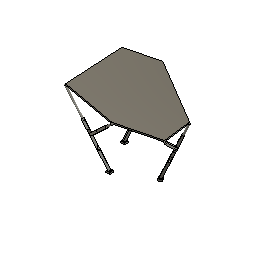
TT-5 (Autodesk Fusion 360 design; units mm, degrees)
Autodesk Fusion 360 part; units mm, degrees
sketch "Sketch1" plane through (0, 0, 0) normal (0, 1, 0) x (1, 0, 0) in component "TT-2 v5 (2)"
  line L0 (2.5, -2.5) -> (-2.5, -2.5)
  line L1 (-2.5, -2.5) -> (-2.5, 2.5)
  line L2 (-2.5, 2.5) -> (2.5, 2.5)
  line L3 (2.5, 2.5) -> (2.5, -2.5)
  constraint horizontal L0
  constraint vertical L1
  constraint horizontal L2
  constraint vertical L3
extrude "Extrude1" add sketch "Sketch1" along normal blind 2.5 makes body 1 in component "TT-2 v5 (2)"
sketch "Sketch2" plane through (0, 0, 0) normal (0, 1, 0) x (1, 0, 0) in component "TT-2 v5 (2)"
  line L0 (1.5, -1.5) -> (-1.5, -1.5)
  line L1 (-1.5, -1.5) -> (-1.5, 1.5)
  line L2 (-1.5, 1.5) -> (1.5, 1.5)
  line L3 (1.5, 1.5) -> (1.5, -1.5)
  constraint horizontal L0
  constraint vertical L1
  constraint horizontal L2
  constraint vertical L3
extrude "Extrude2" add sketch "Sketch2" along normal blind 60 separate body makes body 2 in component "TT-2 v5 (2)"
move_body "Move1" bodies 2 to x (0.939693, -0.34202, 0) y (0.34202, 0.939693, 0) z (0, 0, 1) at (-0.0905, -0.513, 0) in component "TT-2 v5 (2)"
move_body "Move2" bodies 2 to x (1, 0, 0) y (0, 1, 0) z (0, 0, 1) at (3.3727, 9.6612, 0) in component "TT-2 v5 (2)"
sphere "SpherePrimitive1" add diameter 3 placed x (0, 0, 1) y (-0.939693, 0.34202, 0) z (-0.34202, -0.939693, 0) at (3.3241, 9.1329, 0) bodies 2 in component "TT-2 v5 (2)"
sphere "SpherePrimitive2" cut diameter 3 placed x (-1, 0, 0) y (0, 0, 1) z (0, 1, 0) at (0, 2.5, 0) bodies 1 in component "TT-2 v5 (2)"
cylinder "CylinderPrimitive1" add diameter 2.5 height 40 placed x (0.883022, -0.321394, -0.34202) y (-0.321394, 0.116978, -0.939693) z (0.34202, 0.939693, 0) at (23.8453, 65.5145, 0) separate body makes body 3 in component "TT-2 v5 (2)"
sphere "SpherePrimitive3" add diameter 2.5 placed x (0, 0, -1) y (-0.939693, 0.34202, 0) z (0.34202, 0.939693, 0) at (37.5261, 103.1022, 0) bodies 3 in component "TT-2 v5 (2)"
move_body "Move3" bodies 3 2 to x (0.939693, 0.34202, 0) y (-0.34202, 0.939693, 0) z (0, 0, 1) at (23.6283, -3.8286, 0) in component "TT-2 v5 (2)"
move_body "Move4" bodies 2 3 to x (1, 0, 0) y (0, 1, 0) z (0, 0, 1) at (-23.6681, -3.196, 0) in component "TT-2 v5 (2)"
copy_body "CopyPasteBodies1" bodies 3 2 makes body 4 makes body 5 in component "TT-2 v5 (2)"
move_body "Move5" bodies 4 5 to x (1, 0, 0) y (0, 0.906308, 0.422618) z (0, -0.422618, 0.906308) at (0, 42.015, -10.6133) in component "TT-2 v5 (2)"
move_body "Move6" bodies 5 4 to x (1, 0, 0) y (0, 1, 0) z (0, 0, 1) at (0, -2.8403, 9.6134) in component "TT-2 v5 (2)"
extrude "Extrude3" cut 1 faces at (0.4157, 96.2065, 25.0427) along direction (0, -0.906308, -0.422618) blind 15 on bodies 5 bodies 5 in component "TT-2 v5 (2)"
move_body "Move7" bodies 4 to x (1, 0, 0) y (0, 1, 0) z (0, 0, 1) at (0, -26.7116, -12.4558) in component "TT-2 v5 (2)"
move_body "Move8" bodies 5 4 to x (1, 0, 0) y (0, 1, 0) z (0, 0, 1) at (0, -15.5908, 0) in component "TT-2 v5 (2)"
copy_body "CopyPasteBodies2" bodies 4 5 makes body 6 makes body 7 in component "TT-2 v5 (2)"
move_body "Move9" bodies 6 7 to x (0, 0, -1) y (0, 1, 0) z (1, 0, 0) at (-0.0791, 0, -0.06) in component "TT-2 v5 (2)"
move_body "Move10" bodies 6 to x (1, 0, 0) y (0, 1, 0) z (0, 0, 1) at (5.2397, 11.2365, 0) in component "TT-2 v5 (2)"
move_body "Move11" bodies 7 3 4 2 5 6 to x (1, 0, 0) y (0, 0.984808, -0.173648) z (0, 0.173648, 0.984808) at (0, 0.0409, 0.4679) in component "TT-2 v5 (2)"
move_body "Move12" bodies 5 4 to x (1, 0, 0) y (0, 1, 0) z (0, 0, 1) at (0, 17.3834, -3.0131) in component "TT-2 v5 (2)"
sketch "Sketch7" plane through (0, 0, 0) normal (0, 1, 0) x (1, 0, 0) in component "TT-2 v5 (2)"
  line L0 (20, -30) -> (50, 15)
  line L1 (50, 15) -> (20, 47.2574)
  line L2 (20, 47.2574) -> (-26.886, 18.4817)
  line L3 (-26.886, 18.4817) -> (-3.443, -34.2088)
  line L4 (-3.443, -34.2088) -> (20, -30)
extrude "Extrude4" add sketch "Sketch7" along normal blind 2 separate body makes body 8 in component "TT-2 v5 (2)"
move_body "Move13" bodies 8 to x (1, 0, 0) y (0, 1, 0) z (0, 0, 1) at (0, 114.7446, 0) in component "TT-2 v5 (2)"
sketch "Sketch8" plane through (0, 114.7446, 0) normal (0, -1, 0) x (1, 0, 0) in component "TT-2 v5 (2)"
  line L0 (20, 30) -> (-3.443, 34.2088)
  line L1 (-3.443, 34.2088) -> (-26.886, -18.4817)
  line L2 (-26.886, -18.4817) -> (20, -47.2574)
  line L3 (20, -47.2574) -> (50, -15)
  line L4 (50, -15) -> (20, 30)
sphere "SpherePrimitive4" cut diameter 2.5 placed x (1, 0, 0) y (0, 0, 1) z (0, -1, 0) at (-5, 114.7446, -17) bodies 8 in component "TT-2 v5 (2)"
sphere "SpherePrimitive5" cut diameter 2.5 placed x (1, 0, 0) y (0, 0, 1) z (0, -1, 0) at (3, 114.7446, 17) bodies 8 in component "TT-2 v5 (2)"
sphere "SpherePrimitive6" cut diameter 2.5 placed x (1, 0, 0) y (0, 0, 1) z (0, -1, 0) at (32.239, 114.7446, -14.3242) bodies 8 in component "TT-2 v5 (2)"
copy_body "CopyPasteBodies3" bodies 7 5 makes body 9 makes body 10 in component "TT-2 v5 (2)"
extrude "Extrude5" cut 1 faces at (19.5306, 65.7186, -10.5804) along direction (-0.422618, -0.892539, 0.157379) blind 45 on bodies 9 bodies 9 in component "TT-2 v5 (2)"
extrude "Extrude6" cut 1 faces at (-0.5843, 86.4162, 5.2019) along direction (0, -0.965926, -0.258819) blind 45 on bodies 10 bodies 10 in component "TT-2 v5 (2)"
combine "Combine1" operation cut target body 2 tool bodies 9 in component "TT-2 v5 (2)"
combine "Combine2" operation cut target body 2 tool bodies 10 in component "TT-2 v5 (2)"
copy_body "CopyPasteBodies4" bodies 7 5 makes body 11 makes body 12 in component "TT-2 v5 (2)"
combine "Combine3" operation cut target body 2 tool bodies 11 12 in component "TT-2 v5 (2)"
copy_body "Body->Comp1" bodies 1 removing the originals makes body 13 in component "MainFix (2)"
copy_body "Body->Comp2" bodies 3 removing the originals makes body 14 in component "MainAct (2)"
copy_body "Body->Comp3" bodies 4 removing the originals makes body 15 in component "LeftAct (2)"
copy_body "Body->Comp4" bodies 2 removing the originals makes body 16 in component "MainBranch (2)"
copy_body "Body->Comp5" bodies 5 removing the originals makes body 17 in component "LeftBranch (2)"
sketch "Sketch1 (2)" plane through (0, 0, 0) normal (0, 1, 0) x (1, 0, 0) in component "TT-2 v5 (1)"
  line L0 (2.5, -2.5) -> (-2.5, -2.5)
  line L1 (-2.5, -2.5) -> (-2.5, 2.5)
  line L2 (-2.5, 2.5) -> (2.5, 2.5)
  line L3 (2.5, 2.5) -> (2.5, -2.5)
  constraint horizontal L0
  constraint vertical L1
  constraint horizontal L2
  constraint vertical L3
extrude "Extrude1'" add sketch "Sketch1 (2)" along normal blind 2.5 separate body makes body 18 in component "TT-2 v5 (1)"
sketch "Sketch2 (2)" plane through (0, 0, 0) normal (0, 1, 0) x (1, 0, 0) in component "TT-2 v5 (1)"
  line L0 (1.5, -1.5) -> (-1.5, -1.5)
  line L1 (-1.5, -1.5) -> (-1.5, 1.5)
  line L2 (-1.5, 1.5) -> (1.5, 1.5)
  line L3 (1.5, 1.5) -> (1.5, -1.5)
  constraint horizontal L0
  constraint vertical L1
  constraint horizontal L2
  constraint vertical L3
extrude "Extrude2'" add sketch "Sketch2 (2)" along normal blind 60 separate body makes body 19 in component "TT-2 v5 (1)"
move_body "Move1'" bodies 19 to x (0.939693, -0.34202, 0) y (0.34202, 0.939693, 0) z (0, 0, 1) at (-0.0905, -0.513, 0) in component "TT-2 v5 (1)"
move_body "Move2'" bodies 19 to x (1, 0, 0) y (0, 1, 0) z (0, 0, 1) at (3.3727, 9.6612, 0) in component "TT-2 v5 (1)"
sphere "SpherePrimitive1'" add diameter 3 placed x (0, 0, 1) y (-0.939693, 0.34202, 0) z (-0.34202, -0.939693, 0) at (3.3241, 9.1329, 0) bodies 19 in component "TT-2 v5 (1)"
sphere "SpherePrimitive2'" cut diameter 3 placed x (-1, 0, 0) y (0, 0, 1) z (0, 1, 0) at (0, 2.5, 0) bodies 18 in component "TT-2 v5 (1)"
cylinder "CylinderPrimitive1'" add diameter 2.5 height 40 placed x (0.883022, -0.321394, -0.34202) y (-0.321394, 0.116978, -0.939693) z (0.34202, 0.939693, 0) at (23.8453, 65.5145, 0) separate body makes body 20 in component "TT-2 v5 (1)"
sphere "SpherePrimitive3'" add diameter 2.5 placed x (0, 0, -1) y (-0.939693, 0.34202, 0) z (0.34202, 0.939693, 0) at (37.5261, 103.1022, 0) bodies 20 in component "TT-2 v5 (1)"
move_body "Move3'" bodies 20 19 to x (0.939693, 0.34202, 0) y (-0.34202, 0.939693, 0) z (0, 0, 1) at (23.6283, -3.8286, 0) in component "TT-2 v5 (1)"
move_body "Move4'" bodies 19 20 to x (1, 0, 0) y (0, 1, 0) z (0, 0, 1) at (-23.6681, -3.196, 0) in component "TT-2 v5 (1)"
copy_body "CopyPasteBodies1'" bodies 20 19 makes body 21 makes body 22 in component "TT-2 v5 (1)"
move_body "Move5'" bodies 21 22 to x (1, 0, 0) y (0, 0.906308, 0.422618) z (0, -0.422618, 0.906308) at (0, 42.015, -10.6133) in component "TT-2 v5 (1)"
move_body "Move6'" bodies 22 21 to x (1, 0, 0) y (0, 1, 0) z (0, 0, 1) at (0, -2.8403, 9.6134) in component "TT-2 v5 (1)"
extrude "Extrude3'" cut 1 faces at (0.4157, 96.2065, 25.0427) along direction (0, -0.906308, -0.422618) blind 15 on bodies 22 bodies 22 in component "TT-2 v5 (1)"
move_body "Move7'" bodies 21 to x (1, 0, 0) y (0, 1, 0) z (0, 0, 1) at (0, -26.7116, -12.4558) in component "TT-2 v5 (1)"
move_body "Move8'" bodies 22 21 to x (1, 0, 0) y (0, 1, 0) z (0, 0, 1) at (0, -15.5908, 0) in component "TT-2 v5 (1)"
copy_body "CopyPasteBodies2'" bodies 21 22 makes body 23 makes body 24 in component "TT-2 v5 (1)"
move_body "Move9'" bodies 23 24 to x (0, 0, -1) y (0, 1, 0) z (1, 0, 0) at (-0.0791, 0, -0.06) in component "TT-2 v5 (1)"
move_body "Move10'" bodies 23 to x (1, 0, 0) y (0, 1, 0) z (0, 0, 1) at (5.2397, 11.2365, 0) in component "TT-2 v5 (1)"
move_body "Move11'" bodies 24 20 21 19 22 23 to x (1, 0, 0) y (0, 0.984808, -0.173648) z (0, 0.173648, 0.984808) at (0, 0.0409, 0.4679) in component "TT-2 v5 (1)"
move_body "Move12'" bodies 22 21 to x (1, 0, 0) y (0, 1, 0) z (0, 0, 1) at (0, 17.3834, -3.0131) in component "TT-2 v5 (1)"
sketch "Sketch7 (2)" plane through (0, 0, 0) normal (0, 1, 0) x (1, 0, 0) in component "TT-2 v5 (1)"
  line L0 (20, -30) -> (50, 15)
  line L1 (50, 15) -> (20, 47.2574)
  line L2 (20, 47.2574) -> (-26.886, 18.4817)
  line L3 (-26.886, 18.4817) -> (-3.443, -34.2088)
  line L4 (-3.443, -34.2088) -> (20, -30)
extrude "Extrude4'" add sketch "Sketch7 (2)" along normal blind 2 separate body makes body 25 in component "TT-2 v5 (1)"
move_body "Move13'" bodies 25 to x (1, 0, 0) y (0, 1, 0) z (0, 0, 1) at (0, 114.7446, 0) in component "TT-2 v5 (1)"
sketch "Sketch8 (2)" plane through (0, 114.7446, 0) normal (0, -1, 0) x (1, 0, 0) in component "TT-2 v5 (1)"
  line L0 (20, 30) -> (-3.443, 34.2088)
  line L1 (-3.443, 34.2088) -> (-26.886, -18.4817)
  line L2 (-26.886, -18.4817) -> (20, -47.2574)
  line L3 (20, -47.2574) -> (50, -15)
  line L4 (50, -15) -> (20, 30)
sphere "SpherePrimitive4'" cut diameter 2.5 placed x (1, 0, 0) y (0, 0, 1) z (0, -1, 0) at (-5, 114.7446, -17) bodies 25 in component "TT-2 v5 (1)"
sphere "SpherePrimitive5'" cut diameter 2.5 placed x (1, 0, 0) y (0, 0, 1) z (0, -1, 0) at (3, 114.7446, 17) bodies 25 in component "TT-2 v5 (1)"
sphere "SpherePrimitive6'" cut diameter 2.5 placed x (1, 0, 0) y (0, 0, 1) z (0, -1, 0) at (32.239, 114.7446, -14.3242) bodies 25 in component "TT-2 v5 (1)"
copy_body "CopyPasteBodies3'" bodies 24 22 makes body 26 makes body 27 in component "TT-2 v5 (1)"
extrude "Extrude5'" cut 1 faces at (19.5306, 65.7186, -10.5804) along direction (-0.422618, -0.892539, 0.157379) blind 45 on bodies 26 bodies 26 in component "TT-2 v5 (1)"
extrude "Extrude6'" cut 1 faces at (-0.5843, 86.4162, 5.2019) along direction (0, -0.965926, -0.258819) blind 45 on bodies 27 bodies 27 in component "TT-2 v5 (1)"
combine "Combine1'" operation cut target body 19 tool bodies 26 in component "TT-2 v5 (1)"
combine "Combine2'" operation cut target body 19 tool bodies 27 in component "TT-2 v5 (1)"
copy_body "CopyPasteBodies4'" bodies 24 22 makes body 28 makes body 29 in component "TT-2 v5 (1)"
combine "Combine3'" operation cut target body 19 tool bodies 28 29 in component "TT-2 v5 (1)"
copy_body "Body->Comp1'" bodies 18 removing the originals makes body 30 in component "MainFix (1)"
copy_body "Body->Comp2'" bodies 20 removing the originals makes body 31 in component "MainAct (1)"
copy_body "Body->Comp3'" bodies 21 removing the originals makes body 32 in component "LeftAct (1)"
copy_body "Body->Comp4'" bodies 19 removing the originals makes body 33 in component "MainBranch (1)"
copy_body "Body->Comp5'" bodies 22 removing the originals makes body 34 in component "LeftBranch (1)"
sketch "Sketch1 (3)" plane through (0, 0, 0) normal (0, 1, 0) x (1, 0, 0) in component "TT-2 v5"
  line L0 (2.5, -2.5) -> (-2.5, -2.5)
  line L1 (-2.5, -2.5) -> (-2.5, 2.5)
  line L2 (-2.5, 2.5) -> (2.5, 2.5)
  line L3 (2.5, 2.5) -> (2.5, -2.5)
  constraint horizontal L0
  constraint vertical L1
  constraint horizontal L2
  constraint vertical L3
extrude "Extrude1''" add sketch "Sketch1 (3)" along normal blind 2.5 separate body makes body 35 in component "TT-2 v5"
sketch "Sketch2 (3)" plane through (0, 0, 0) normal (0, 1, 0) x (1, 0, 0) in component "TT-2 v5"
  line L0 (1.5, -1.5) -> (-1.5, -1.5)
  line L1 (-1.5, -1.5) -> (-1.5, 1.5)
  line L2 (-1.5, 1.5) -> (1.5, 1.5)
  line L3 (1.5, 1.5) -> (1.5, -1.5)
  constraint horizontal L0
  constraint vertical L1
  constraint horizontal L2
  constraint vertical L3
extrude "Extrude2''" add sketch "Sketch2 (3)" along normal blind 60 separate body makes body 36 in component "TT-2 v5"
move_body "Move1''" bodies 36 to x (0.939693, -0.34202, 0) y (0.34202, 0.939693, 0) z (0, 0, 1) at (-0.0905, -0.513, 0) in component "TT-2 v5"
move_body "Move2''" bodies 36 to x (1, 0, 0) y (0, 1, 0) z (0, 0, 1) at (3.3727, 9.6612, 0) in component "TT-2 v5"
sphere "SpherePrimitive1''" add diameter 3 placed x (0, 0, 1) y (-0.939693, 0.34202, 0) z (-0.34202, -0.939693, 0) at (3.3241, 9.1329, 0) bodies 36 in component "TT-2 v5"
sphere "SpherePrimitive2''" cut diameter 3 placed x (-1, 0, 0) y (0, 0, 1) z (0, 1, 0) at (0, 2.5, 0) bodies 35 in component "TT-2 v5"
cylinder "CylinderPrimitive1''" add diameter 2.5 height 40 placed x (0.883022, -0.321394, -0.34202) y (-0.321394, 0.116978, -0.939693) z (0.34202, 0.939693, 0) at (23.8453, 65.5145, 0) separate body makes body 37 in component "TT-2 v5"
sphere "SpherePrimitive3''" add diameter 2.5 placed x (0, 0, -1) y (-0.939693, 0.34202, 0) z (0.34202, 0.939693, 0) at (37.5261, 103.1022, 0) bodies 37 in component "TT-2 v5"
move_body "Move3''" bodies 37 36 to x (0.939693, 0.34202, 0) y (-0.34202, 0.939693, 0) z (0, 0, 1) at (23.6283, -3.8286, 0) in component "TT-2 v5"
move_body "Move4''" bodies 36 37 to x (1, 0, 0) y (0, 1, 0) z (0, 0, 1) at (-23.6681, -3.196, 0) in component "TT-2 v5"
copy_body "CopyPasteBodies1''" bodies 37 36 makes body 38 makes body 39 in component "TT-2 v5"
move_body "Move5''" bodies 38 39 to x (1, 0, 0) y (0, 0.906308, 0.422618) z (0, -0.422618, 0.906308) at (0, 42.015, -10.6133) in component "TT-2 v5"
move_body "Move6''" bodies 39 38 to x (1, 0, 0) y (0, 1, 0) z (0, 0, 1) at (0, -2.8403, 9.6134) in component "TT-2 v5"
extrude "Extrude3''" cut 1 faces at (0.4157, 96.2065, 25.0427) along direction (0, -0.906308, -0.422618) blind 15 on bodies 39 bodies 39 in component "TT-2 v5"
move_body "Move7''" bodies 38 to x (1, 0, 0) y (0, 1, 0) z (0, 0, 1) at (0, -26.7116, -12.4558) in component "TT-2 v5"
move_body "Move8''" bodies 39 38 to x (1, 0, 0) y (0, 1, 0) z (0, 0, 1) at (0, -15.5908, 0) in component "TT-2 v5"
copy_body "CopyPasteBodies2''" bodies 38 39 makes body 40 makes body 41 in component "TT-2 v5"
move_body "Move9''" bodies 40 41 to x (0, 0, -1) y (0, 1, 0) z (1, 0, 0) at (-0.0791, 0, -0.06) in component "TT-2 v5"
move_body "Move10''" bodies 40 to x (1, 0, 0) y (0, 1, 0) z (0, 0, 1) at (5.2397, 11.2365, 0) in component "TT-2 v5"
move_body "Move11''" bodies 41 37 38 36 39 40 to x (1, 0, 0) y (0, 0.984808, -0.173648) z (0, 0.173648, 0.984808) at (0, 0.0409, 0.4679) in component "TT-2 v5"
move_body "Move12''" bodies 39 38 to x (1, 0, 0) y (0, 1, 0) z (0, 0, 1) at (0, 17.3834, -3.0131) in component "TT-2 v5"
sketch "Sketch7 (3)" plane through (0, 0, 0) normal (0, 1, 0) x (1, 0, 0) in component "TT-2 v5"
  line L0 (20, -30) -> (50, 15)
  line L1 (50, 15) -> (20, 47.2574)
  line L2 (20, 47.2574) -> (-26.886, 18.4817)
  line L3 (-26.886, 18.4817) -> (-3.443, -34.2088)
  line L4 (-3.443, -34.2088) -> (20, -30)
extrude "Extrude4''" add sketch "Sketch7 (3)" along normal blind 2 separate body makes body 42 in component "TT-2 v5"
move_body "Move13''" bodies 42 to x (1, 0, 0) y (0, 1, 0) z (0, 0, 1) at (0, 114.7446, 0) in component "TT-2 v5"
sketch "Sketch8 (3)" plane through (0, 114.7446, 0) normal (0, -1, 0) x (1, 0, 0) in component "TT-2 v5"
  line L0 (20, 30) -> (-3.443, 34.2088)
  line L1 (-3.443, 34.2088) -> (-26.886, -18.4817)
  line L2 (-26.886, -18.4817) -> (20, -47.2574)
  line L3 (20, -47.2574) -> (50, -15)
  line L4 (50, -15) -> (20, 30)
sphere "SpherePrimitive4''" cut diameter 2.5 placed x (1, 0, 0) y (0, 0, 1) z (0, -1, 0) at (-5, 114.7446, -17) bodies 42 in component "TT-2 v5"
sphere "SpherePrimitive5''" cut diameter 2.5 placed x (1, 0, 0) y (0, 0, 1) z (0, -1, 0) at (3, 114.7446, 17) bodies 42 in component "TT-2 v5"
sphere "SpherePrimitive6''" cut diameter 2.5 placed x (1, 0, 0) y (0, 0, 1) z (0, -1, 0) at (32.239, 114.7446, -14.3242) bodies 42 in component "TT-2 v5"
copy_body "CopyPasteBodies3''" bodies 41 39 makes body 43 makes body 44 in component "TT-2 v5"
extrude "Extrude5''" cut 1 faces at (19.5306, 65.7186, -10.5804) along direction (-0.422618, -0.892539, 0.157379) blind 45 on bodies 43 bodies 43 in component "TT-2 v5"
extrude "Extrude6''" cut 1 faces at (-0.5843, 86.4162, 5.2019) along direction (0, -0.965926, -0.258819) blind 45 on bodies 44 bodies 44 in component "TT-2 v5"
combine "Combine1''" operation cut target body 36 tool bodies 43 in component "TT-2 v5"
combine "Combine2''" operation cut target body 36 tool bodies 44 in component "TT-2 v5"
copy_body "CopyPasteBodies4''" bodies 41 39 makes body 45 makes body 46 in component "TT-2 v5"
combine "Combine3''" operation cut target body 36 tool bodies 45 46 in component "TT-2 v5"
copy_body "Body->Comp1''" bodies 35 removing the originals makes body 47 in component "MainFix"
copy_body "Body->Comp2''" bodies 37 removing the originals makes body 48 in component "MainAct"
copy_body "Body->Comp3''" bodies 38 removing the originals makes body 49 in component "LeftAct"
copy_body "Body->Comp4''" bodies 36 removing the originals makes body 50 in component "MainBranch"
copy_body "Body->Comp5''" bodies 39 removing the originals makes body 51 in component "LeftBranch"
sketch "Sketch1 (4)" plane through (0, 0, 0) normal (0, 1, 0) x (1, 0, 0)
  line L0 (60, -50) -> (100, -10)
  line L1 (100, -10) -> (80, 23.8601)
  line L2 (80, 23.8601) -> (-14.3851, 31.448)
  line L3 (-14.3851, 31.448) -> (-45.4952, 0.3378)
  line L4 (-45.4952, 0.3378) -> (-8.0113, -72.9607)
  line L5 (-8.0113, -72.9607) -> (60, -50)
  constraint parallel L0 L3
extrude "Extrude1'''" add sketch "Sketch1 (4)" along normal blind 2 separate body makes body 52
move_body "Move1'''" bodies 52 to x (1, 0, 0) y (0, 1, 0) z (0, 0, 1) at (0, 98.4044, 0)
copy_body "Body->Comp1'''" bodies 52 removing the originals makes body 53 in component "Component"
component "TT-4 v2 (2)" placed x (1, 0, 0) y (0, 1, 0) z (0, 0, 1) at (0, 0, 0)
component "TT-4 v2 (1)" placed x (0.5, 0, 0.866025) y (0, 1, 0) z (-0.866025, 0, 0.5) at (69.4304, 0, 19.3881)
component "TT-4 v2" placed x (-0.064221, 0, -0.997936) y (0, 1, 0) z (0.997936, 0, -0.064221) at (25.4418, 0, 45.9838)
component "Component" placed x (1, 0, 0) y (0, 1, 0) z (0, 0, 1) at (0, 0, 0)
component "TT-2 v5" placed x (1, 0, 0) y (0, 1, 0) z (0, 0, 1) at (0, 0, 0) in component "TT-4 v2"
component "MainFix" placed x (1, 0, 0) y (0, 1, 0) z (0, 0, 1) at (0, 0, 0) in component "TT-2 v5"
component "MainAct" placed x (-0.13462, 0.309445, 0.94134) y (-0.399324, 0.85249, -0.337344) z (-0.906873, -0.421313, 0.008806) at (-0.1242, 4.8498, -0.7952) in component "TT-2 v5"
component "LeftAct" placed x (0.110637, -0.633904, 0.765458) y (0.303111, 0.755014, 0.581444) z (-0.946511, 0.16769, 0.275675) at (-29.2097, 12.5203, -33.521) in component "TT-2 v5"
component "MainBranch" placed x (-0.13462, 0.309445, 0.94134) y (-0.399324, 0.85249, -0.337344) z (-0.906873, -0.421313, 0.008806) at (1.0706, 0.2153, 0.9465) in component "TT-2 v5"
component "LeftBranch" placed x (0.110637, -0.633904, 0.765458) y (0.303111, 0.755014, 0.581444) z (-0.946511, 0.16769, 0.275675) at (-29.4544, 8.4575, -36.7921) in component "TT-2 v5"
component "TT-2 v5 (1)" placed x (1, 0, 0) y (0, 1, 0) z (0, 0, 1) at (0, 0, 0) in component "TT-4 v2 (1)"
component "MainFix (1)" placed x (1, 0, 0) y (0, 1, 0) z (0, 0, 1) at (0, 0, 0) in component "TT-2 v5 (1)"
component "MainAct (1)" placed x (0.859708, 0.392723, 0.326606) y (-0.37056, 0.919613, -0.130371) z (-0.35155, -0.008946, 0.936126) at (-0.7482, 5.2226, -1.3187) in component "TT-2 v5 (1)"
component "LeftAct (1)" placed x (-0.635171, -0.042868, -0.771181) y (0.108693, 0.983561, -0.144198) z (0.764685, -0.175412, -0.62007) at (-13.6185, -8.9853, -8.1408) in component "TT-2 v5 (1)"
component "MainBranch (1)" placed x (0.859708, 0.392723, 0.326606) y (-0.37056, 0.919613, -0.130371) z (-0.35155, -0.008946, 0.936126) at (1.0327, 0.0378, 0.3643) in component "TT-2 v5 (1)"
component "LeftBranch (1)" placed x (-0.635171, -0.042868, -0.771181) y (0.108693, 0.983561, -0.144198) z (0.764685, -0.175412, -0.62007) at (-11.9393, -3.8877, -9.865) in component "TT-2 v5 (1)"
component "TT-2 v5 (2)" placed x (1, 0, 0) y (0, 1, 0) z (0, 0, 1) at (0, 0, 0) in component "TT-4 v2 (2)"
component "MainFix (2)" placed x (1, 0, 0) y (0, 1, 0) z (0, 0, 1) at (0, 0, 0) in component "TT-2 v5 (2)"
component "MainAct (2)" placed x (0.977956, 0.180595, 0.104822) y (-0.165333, 0.976313, -0.13956) z (-0.127543, 0.119153, 0.98465) at (0.1667, 1.7019, -0.2255) in component "TT-2 v5 (2)"
component "LeftAct (2)" placed x (0.824256, 0.565818, 0.021247) y (-0.562107, 0.822211, -0.089472) z (-0.068094, 0.061805, 0.995763) at (17.8167, 6.2949, -1.6653) in component "TT-2 v5 (2)"
component "MainBranch (2)" placed x (0.977956, 0.180595, 0.104822) y (-0.165333, 0.976313, -0.13956) z (-0.127543, 0.119153, 0.98465) at (0.4844, -0.1235, 0.3802) in component "TT-2 v5 (2)"
component "LeftBranch (2)" placed x (0.824256, 0.565818, 0.021247) y (-0.562107, 0.822211, -0.089472) z (-0.068094, 0.061805, 0.995763) at (17.9828, 6.1331, -1.7039) in component "TT-2 v5 (2)"
hidden bodies 40 41 42 23 24 25 7 6 8
named bodies: "MainFix", "MainBranch", "MainAct", "LeftAct", "LeftBranch", "MainAct (1)", "MainBranch (1)", "RightAct", "RightBranch", "Flat", "RightBranch (1)", "LeftBranch (1)"
